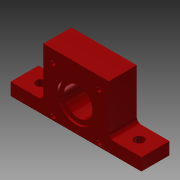
# Autodesk Inventor part: Igus Bracket
Saved by Autodesk Inventor 2014 (Build 180170000, 170)
## iProperties
Created: 2014-01-17
Part Number: Igus Bracket
Material: Generic
Document SubType Name: Modeling
Designer: PLTW
Density: 1 g/cm^3
Appearance: Red
Author: PLTW
Autodesk Inventor part; units mm, degrees
ref_plane "YZ Plane" through (0, 0, 0) normal (1, 0, 0) x (0, 1, 0)
ref_plane "XZ Plane" through (0, 0, 0) normal (0, 1, 0) x (-1, 0, 0)
ref_plane "XY Plane" through (0, 0, 0) normal (0, 0, 1) x (1, 0, 0)
sketch "Sketch1" plane through (0, 0, 0) normal (0, 0, 1) x (1, 0, 0)
  circle A0 centre (0, 0) radius 9.6393
  line L0 (-44.45, -18.0213) -> (44.45, -18.0213)
  line L1 (-44.45, -18.0213) -> (-44.45, -9.6393)
  line L2 (-44.45, -9.6393) -> (-22.225, -9.6393)
  line L3 (44.45, -18.0213) -> (44.45, -9.6393)
  line L4 (44.45, -9.6393) -> (22.225, -9.6393)
  line L5 (22.225, -9.6393) -> (22.225, 23.8887)
  line L6 (22.225, 23.8887) -> (-22.225, 23.8887)
  line L7 (-22.225, 23.8887) -> (-22.225, -9.6393)
  point P0 (0, -18.0213)
  dimension "d0" = 19.2786
  dimension "d1" = 88.9
  dimension "d3" = 8.382
  dimension "d16" = 44.45
  dimension "d17" = 41.91
  dimension "d18" = 18.0213
  constraints: 16 end point, 4 perpendicular, 2 horizontal, 1 centre point, 1 coincident, 1 collinear, 1 horizontal alignment, 1 midpoint, 1 parallel, 1 vertical, 1 vertical alignment
  measures "d0" diameter of A0
  measures "d1" distance of L0.start L0.end
  measures "d3" distance of L0.start L1.end
  measures "d16" distance of L5.end L6.end
  measures "d17" distance between parallel lines of L0 L6
  measures "d18" distance of point (0, -18.021) point (0, 0)
extrude "Extrusion1" add sketch "Sketch1" along normal blind 19.05
sketch "Sketch2" plane through (22.225, -9.6393, 0) normal (0, 1, 0) x (1, 0, 0)
  line L0 (22.225, 0) -> (0, 0) projected
  line L1 (22.225, 0) -> (22.225, -19.05) projected
  line L2 (-44.45, 0) -> (-66.675, 0) projected
  line L3 (-66.675, 0) -> (-66.675, -19.05) projected
  line L4 (-44.45, -19.05) -> (-66.675, -19.05) projected
  line L5 (-44.45, 0) -> (-44.45, -19.05) projected
  circle A0 centre (-55.5625, -9.525) radius 3.175
  circle A1 centre (11.1125, -9.525) radius 3.175
  point P0 (-22.225, 0)
  point P1 (11.1125, 0)
  point P2 (-55.5625, 0)
  point P3 (22.225, -9.525)
  dimension "d8" = 6.35
  constraints: 3 midpoint, 2 centre point, 2 horizontal alignment, 2 vertical alignment, 1 equal radius
  measures "d8" diameter of A0
extrude "Extrusion2" cut sketch "Sketch2" against normal through all contours A0 | A1
fillet "Fillet1" radius 3.175 2 edges at (22.225, -9.6393, 9.525) (-22.225, -9.6393, 9.525)
sketch "Sketch3" plane through (0, 0, 19.05) normal (0, 0, 1) x (1, 0, 0)
  circle A0 centre (0, 0) radius 9.6393 projected
  circle A1 centre (0, 0) radius 12.7
  dimension "d12" = 25.4
  constraints: 1 centre point, 1 coincident
  measures "d12" diameter of A1
extrude "Extrusion3" cut sketch "Sketch3" against normal blind 1.524
sketch "Sketch4" plane through (0, 0, 0) normal (0, 0, -1) x (-1, 0, 0)
  circle A0 centre (15.5335, 15.5335) radius 1.5 projected
  circle A1 centre (-15.5335, 15.5335) radius 1.5 projected
  circle A2 centre (15.5335, -15.5335) radius 1.5 projected
  circle A3 centre (-15.5335, -15.5335) radius 1.5 projected
extrude "Extrusion4" cut sketch "Sketch4" against normal through all
sketch "Sketch5" plane through (0, 0, 0) normal (0, 0, -1) x (-1, 0, 0)
  circle A0 centre (15.5335, -15.5335) radius 1.5 projected
  circle A1 centre (15.5335, 15.5335) radius 1.5 projected
  circle A2 centre (-15.5335, 15.5335) radius 1.5 projected
  circle A3 centre (-15.5335, -15.5335) radius 1.5 projected
  circle A4 centre (-15.5335, 15.5335) radius 3.81
  circle A5 centre (15.5335, 15.5335) radius 3.81
  circle A6 centre (-15.5335, -15.5335) radius 3.81
  circle A7 centre (15.5335, -15.5335) radius 3.81
  dimension "d21" = 7.62
  constraints: 4 centre point, 4 coincident, 3 equal radius
  measures "d21" diameter of A4
ref_plane "Work Plane1" through (-24.1011, -23.3184, -29.3654) normal (0, 0, 1) x (1, 0, 0)
extrude "Extrusion5" add sketch "Sketch5" along normal up to surface (29.3654 mm away)
sketch "Sketch6" plane through (0, 0, 19.05) normal (0, 0, 1) x (1, 0, 0)
  line L0 (-44.45, -18.0213) -> (44.45, -18.0213) projected
  line L1 (-34.925, -18.0213) -> (32.5275, -18.0213)
  line L2 (32.5275, -18.0213) -> (32.5275, -39.2458)
  line L3 (32.5275, -39.2458) -> (-34.925, -39.2458)
  line L4 (-34.925, -39.2458) -> (-34.925, -18.0213)
  constraints: 8 end point, 2 parallel, 1 horizontal, 1 perpendicular, 1 point on line
extrude "Extrusion6" cut sketch "Sketch6" against normal through all
fillet "Fillet2" radius 12.7 2 edges at (22.225, 23.8887, 9.525) (-22.225, 23.8887, 9.525)
body "Solid1"
